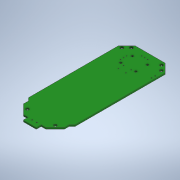
# Autodesk Inventor part: PCB
Saved by Autodesk Inventor 2020 (Build 240168000, 168)
## iProperties
Created: 2021-01-14
Part Number: PCB
Material: Generic
Document SubType Name: Modeling
Designer: Luke
Density: 1 g/cm^3
Appearance: Default
Author: Luke
Autodesk Inventor part; units mm, degrees
ref_plane "YZ Plane" through (0, 0, 0) normal (1, 0, 0) x (0, 1, 0)
ref_plane "XZ Plane" through (0, 0, 0) normal (0, 1, 0) x (-1, 0, 0)
ref_plane "XY Plane" through (0, 0, 0) normal (0, 0, 1) x (1, 0, 0)
sketch "Sketch1" plane through (0, 0, 0) normal (0, 1, 0) x (-1, 0, 0)
  line L0 (5.5496, 46.5995) -> (5.5496, 50.3655)
  arc A0 (5.5496, 50.3655) -> (5.2006, 50.7145) centre (5.2006, 50.3655) ccw
  line L1 (5.2006, 50.7145) -> (-5.2234, 50.7145)
  arc A1 (-5.2234, 50.7145) -> (-5.4614, 50.4765) centre (-5.2234, 50.4765) ccw
  line L2 (-5.4614, 50.4765) -> (-5.4614, 46.5995)
  line L3 (-5.4614, 46.5995) -> (-9.2444, 46.5995)
  line L4 (-9.2444, 46.5995) -> (-17.2394, 38.6045)
  line L5 (-17.2394, 38.6045) -> (-17.2394, 34.8415)
  line L6 (-17.2394, 34.8415) -> (-19.7395, 32.2255)
  line L7 (-19.7395, 32.2255) -> (-19.7395, -43.6601)
  line L8 (-19.7395, -43.6601) -> (-12.6739, -50.7145)
  line L9 (-12.6739, -50.7145) -> (12.6966, -50.7145)
  line L10 (12.6966, -50.7145) -> (19.6766, -43.7345)
  line L11 (19.6766, -43.7345) -> (19.6766, 32.1505)
  line L12 (19.6766, 32.1505) -> (17.2796, 34.5475)
  line L13 (17.2796, 34.5475) -> (17.2796, 38.6115)
  line L14 (17.2796, 38.6115) -> (9.2916, 46.5995)
  line L15 (9.2916, 46.5995) -> (5.5496, 46.5995)
  circle A2 centre (12.7766, -47.6345) radius 1.27
  circle A3 centre (-12.6044, -47.6345) radius 1.27
  circle A4 centre (16.7766, -43.6345) radius 1.27
  circle A5 centre (-16.4774, -43.6345) radius 1.27
  circle A6 centre (11.7766, 40.9591) radius 1.27
  circle A7 centre (-11.7154, 40.9591) radius 1.27
  circle A8 centre (-1.8694, 46.7845) radius 0.425
  circle A9 centre (1.9306, 46.7845) radius 0.425
  circle A10 centre (-17.8584, -37.1345) radius 0.45
  circle A11 centre (-17.8584, -34.1345) radius 0.45
  arc A12 (3.4251, -26.9975) -> (2.7461, -26.9975) centre (3.0856, -26.9975) ccw
  arc A13 (2.7461, -26.9975) -> (3.4251, -26.9975) centre (3.0856, -26.9975) ccw
  arc A14 (3.4251, -26.9975) -> (2.7461, -26.9975) centre (3.0856, -26.9975) ccw
  arc A15 (2.7461, -26.9975) -> (3.4251, -26.9975) centre (3.0856, -26.9975) ccw
  arc A16 (3.4251, -31.4425) -> (2.7461, -31.4425) centre (3.0856, -31.4425) ccw
  arc A17 (2.7461, -31.4425) -> (3.4251, -31.4425) centre (3.0856, -31.4425) ccw
  arc A18 (3.4251, -31.4425) -> (2.7461, -31.4425) centre (3.0856, -31.4425) ccw
  arc A19 (2.7461, -31.4425) -> (3.4251, -31.4425) centre (3.0856, -31.4425) ccw
  arc A20 (-2.9249, -31.4425) -> (-3.6039, -31.4425) centre (-3.2644, -31.4425) ccw
  arc A21 (-3.6039, -31.4425) -> (-2.9249, -31.4425) centre (-3.2644, -31.4425) ccw
  arc A22 (-2.9249, -31.4425) -> (-3.6039, -31.4425) centre (-3.2644, -31.4425) ccw
  arc A23 (-3.6039, -31.4425) -> (-2.9249, -31.4425) centre (-3.2644, -31.4425) ccw
  arc A24 (-2.9249, -26.9975) -> (-3.6039, -26.9975) centre (-3.2644, -26.9975) ccw
  arc A25 (-3.6039, -26.9975) -> (-2.9249, -26.9975) centre (-3.2644, -26.9975) ccw
  arc A26 (-2.9249, -26.9975) -> (-3.6039, -26.9975) centre (-3.2644, -26.9975) ccw
  arc A27 (-3.6039, -26.9975) -> (-2.9249, -26.9975) centre (-3.2644, -26.9975) ccw
  line L16 (7.0146, -32.9585) -> (7.0146, -31.4505)
  line L17 (7.0146, -31.4505) -> (5.5066, -31.4505)
  line L18 (5.5066, -31.4505) -> (5.5066, -32.9585)
  line L19 (5.5066, -32.9585) -> (7.0146, -32.9585)
  line L20 (7.0146, -32.9585) -> (7.0146, -31.4505)
  line L21 (7.0146, -31.4505) -> (5.5066, -31.4505)
  line L22 (5.5066, -31.4505) -> (5.5066, -32.9585)
  line L23 (5.5066, -32.9585) -> (7.0146, -32.9585)
  line L24 (7.0146, -42.7375) -> (7.0146, -41.2295)
  line L25 (7.0146, -41.2295) -> (5.5066, -41.2295)
  line L26 (5.5066, -41.2295) -> (5.5066, -42.7375)
  line L27 (5.5066, -42.7375) -> (7.0146, -42.7375)
  line L28 (7.0146, -42.7375) -> (7.0146, -41.2295)
  line L29 (7.0146, -41.2295) -> (5.5066, -41.2295)
  line L30 (5.5066, -41.2295) -> (5.5066, -42.7375)
  line L31 (5.5066, -42.7375) -> (7.0146, -42.7375)
  line L32 (-5.6854, -42.7375) -> (-5.6854, -41.2295)
  line L33 (-5.6854, -41.2295) -> (-7.1934, -41.2295)
  line L34 (-7.1934, -41.2295) -> (-7.1934, -42.7375)
  line L35 (-7.1934, -42.7375) -> (-5.6854, -42.7375)
  line L36 (-5.6854, -42.7375) -> (-5.6854, -41.2295)
  line L37 (-5.6854, -41.2295) -> (-7.1934, -41.2295)
  line L38 (-7.1934, -41.2295) -> (-7.1934, -42.7375)
  line L39 (-7.1934, -42.7375) -> (-5.6854, -42.7375)
  line L40 (-5.6854, -32.9585) -> (-5.6854, -31.4505)
  line L41 (-5.6854, -31.4505) -> (-7.1934, -31.4505)
  line L42 (-7.1934, -31.4505) -> (-7.1934, -32.9585)
  line L43 (-7.1934, -32.9585) -> (-5.6854, -32.9585)
  line L44 (-5.6854, -32.9585) -> (-5.6854, -31.4505)
  line L45 (-5.6854, -31.4505) -> (-7.1934, -31.4505)
  line L46 (-7.1934, -31.4505) -> (-7.1934, -32.9585)
  line L47 (-7.1934, -32.9585) -> (-5.6854, -32.9585)
  arc A28 (9.1401, -34.554) -> (8.4611, -34.554) centre (8.8006, -34.554) ccw
  arc A29 (8.4611, -34.554) -> (9.1401, -34.554) centre (8.8006, -34.554) ccw
  arc A30 (9.1401, -34.554) -> (8.4611, -34.554) centre (8.8006, -34.554) ccw
  arc A31 (8.4611, -34.554) -> (9.1401, -34.554) centre (8.8006, -34.554) ccw
  arc A32 (9.1401, -39.634) -> (8.4611, -39.634) centre (8.8006, -39.634) ccw
  arc A33 (8.4611, -39.634) -> (9.1401, -39.634) centre (8.8006, -39.634) ccw
  arc A34 (9.1401, -39.634) -> (8.4611, -39.634) centre (8.8006, -39.634) ccw
  arc A35 (8.4611, -39.634) -> (9.1401, -39.634) centre (8.8006, -39.634) ccw
  arc A36 (9.1401, -37.094) -> (8.4611, -37.094) centre (8.8006, -37.094) ccw
  arc A37 (8.4611, -37.094) -> (9.1401, -37.094) centre (8.8006, -37.094) ccw
  arc A38 (9.1401, -37.094) -> (8.4611, -37.094) centre (8.8006, -37.094) ccw
  arc A39 (8.4611, -37.094) -> (9.1401, -37.094) centre (8.8006, -37.094) ccw
  arc A40 (2.7901, -45.984) -> (2.1111, -45.984) centre (2.4506, -45.984) ccw
  arc A41 (2.1111, -45.984) -> (2.7901, -45.984) centre (2.4506, -45.984) ccw
  arc A42 (2.7901, -45.984) -> (2.1111, -45.984) centre (2.4506, -45.984) ccw
  arc A43 (2.1111, -45.984) -> (2.7901, -45.984) centre (2.4506, -45.984) ccw
  arc A44 (-2.2899, -45.984) -> (-2.9689, -45.984) centre (-2.6294, -45.984) ccw
  arc A45 (-2.9689, -45.984) -> (-2.2899, -45.984) centre (-2.6294, -45.984) ccw
  arc A46 (-2.2899, -45.984) -> (-2.9689, -45.984) centre (-2.6294, -45.984) ccw
  arc A47 (-2.9689, -45.984) -> (-2.2899, -45.984) centre (-2.6294, -45.984) ccw
  arc A48 (0.2501, -45.984) -> (-0.4289, -45.984) centre (-0.0894, -45.984) ccw
  arc A49 (-0.4289, -45.984) -> (0.2501, -45.984) centre (-0.0894, -45.984) ccw
  arc A50 (0.2501, -45.984) -> (-0.4289, -45.984) centre (-0.0894, -45.984) ccw
  arc A51 (-0.4289, -45.984) -> (0.2501, -45.984) centre (-0.0894, -45.984) ccw
  point P0 (5.5496, 50.3655)
  point P1 (-0.4289, -45.984)
  point P2 (0.2501, -45.984)
  point P3 (2.1111, -45.984)
  point P4 (2.7901, -45.984)
  point P5 (8.4611, -39.634)
  point P6 (9.1401, -39.634)
  point P7 (-3.6039, -26.9975)
  point P8 (-2.9249, -26.9975)
  point P9 (2.7461, -31.4425)
  point P10 (3.4251, -31.4425)
  point P11 (2.7461, -26.9975)
  point P12 (3.4251, -26.9975)
  point P13 (-3.6039, -31.4425)
  point P14 (-2.9249, -31.4425)
  point P15 (8.4611, -34.554)
  point P16 (9.1401, -34.554)
  point P17 (8.4611, -37.094)
  point P18 (9.1401, -37.094)
  point P19 (-2.9689, -45.984)
  point P20 (-2.2899, -45.984)
  constraints: 96 end point, 84 point on circle, 52 centre point
extrude "Extrusion1" add sketch "Sketch1" along normal blind 1.23
ref_plane "Work Plane1" through (0, 0.615, 0) normal (0, 1, 0) x (1, 0, 0)
ref_plane "Work Plane3" through (0.0314, 0, 32.2255) normal (1, 0, 0) x (0, 0, -1)
ref_plane "Work Plane5" through (12.6739, 1.23, -50.7145) normal (0, 0.7071068, -0.7071068) x (-1, 0, 0)
body "Solid1"
